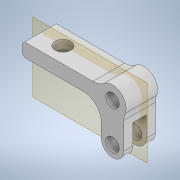
# Autodesk Inventor part: 1번부품
Saved by Autodesk Inventor 2022 (Build 260153000, 153)
## iProperties
Created: 2021-09-05
Part Number: 1번부품
Material: 일반
Document SubType Name: Modeling
Designer: 서울공업고등학교
Density: 1 g/cm^3
Appearance: 기본값
Author: 서울공업고등학교
Autodesk Inventor part; units mm, degrees
ref_plane "YZ Plane" through (0, 0, 0) normal (1, 0, 0) x (0, 1, 0)
ref_plane "XZ Plane" through (0, 0, 0) normal (0, 1, 0) x (-1, 0, 0)
ref_plane "XY Plane" through (0, 0, 0) normal (0, 0, 1) x (1, 0, 0)
sketch "스케치1" plane through (0, 0, 0) normal (0, 0, 1) x (1, 0, 0)
  circle A0 centre (0, 0) radius 3
  arc A1 (-5, 0) -> (5, 0) centre (0, 0) ccw
  circle A2 centre (0, 17) radius 3
  line L0 (-5, 0) -> (8.6834, 0) construction
  line L1 (-40, 14) -> (-40, 20)
  line L2 (-40, 20) -> (-5.1962, 20)
  line L3 (5, 0) -> (5, 13.6834)
  line L4 (-40, 14) -> (-5, 14)
  line L5 (-5, 0) -> (-5, 14)
  arc A3 (5, 13.6834) -> (-5.1962, 20) centre (0, 17) ccw
  dimension "d2" = 6
  dimension "d4" = 17
  dimension "d5" = 10
  dimension "d7" = 6
  dimension "d9" = 6
  dimension "d10" = 40
  dimension "d12" = 14
  dimension "d13" = 6
  constraints: 12 end point, 4 centre point, 4 point on circle, 3 coincident, 2 horizontal, 2 tangent, 2 vertical, 1 parallel, 1 perpendicular, 1 vertical alignment
  measures "d2" diameter of A0
  measures "d4" distance of point (0, 0) A3.centre
  measures "d5" diameter of A1
  measures "d7" diameter of A2
  measures "d9" distance of L1.start L1.end
  measures "d10" distance from line of L1 A3.centre
  measures "d12" distance from line of point (0, 0) L4
  measures "d13" radius of A3
extrude "돌출1" add sketch "스케치1" along normal mid plane 14
chamfer "모따기1" distance 1 angle 45 2 edges at (-40, 20, 0) (-40, 14, 0)
fillet "모깎기1" radius 8 3 edges at (-5, 14, 0) (-5.1962, 20, 0) (5, 13.6834, 0)
sketch "스케치2" plane through (-39, 20, 7) normal (0, 1, 0) x (1, 0, 0)
  circle A0 centre (10, 7) radius 3.5
  line L0 (0, 0) -> (0, 14) projected
  line L1 (30.3397, 0) -> (0, 0) projected
  point P0 (39, 7)
  dimension "d20" = 7
  dimension "d21" = 10
  dimension "d22" = 7
  constraints: 1 centre point
  measures "d20" diameter of A0
  measures "d21" distance from line of L0 A0.centre
  measures "d22" distance from line of A0.centre L1
extrude "돌출2" cut sketch "스케치2" against normal blind 4
ref_plane "작업 평면1" through (0, 0, 0) normal (0, 0, 1) x (1, 0, 0)
sketch "스케치3" plane through (0, 0, 0) normal (0, 0, 1) x (1, 0, 0)
  line L0 (15.6771, 9) -> (-15.3905, 9)
  line L1 (-15.3905, 9) -> (-15.3905, -8.77)
  line L2 (-15.3905, -8.77) -> (15.6771, -8.77)
  line L3 (15.6771, -8.77) -> (15.6771, 9)
  arc A0 (-5, 0) -> (5, 0) centre (0, 0) ccw projected
  dimension "d25" = 14
  constraints: 8 end point, 2 parallel, 1 horizontal, 1 perpendicular
extrude "돌출3" cut sketch "스케치3" along normal mid plane 6
sketch "스케치4" plane through (-39, 20, 7) normal (0, 1, 0) x (1, 0, 0)
  point P0 (39, 7)
